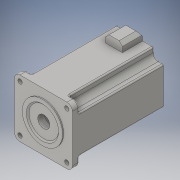
# Autodesk Inventor part: Body
Saved by Autodesk Inventor 2016 (Build 200138000, 138)
## iProperties
Created: 2017-05-16
Part Number: Body
Material: Generic
Document SubType Name: Modeling
Designer: M220404
Density: 1 g/cm^3
Appearance: Default
Author: M220404
Autodesk Inventor part; units mm, degrees
ref_plane "YZ Plane" through (0, 0, 0) normal (1, 0, 0) x (0, 1, 0)
ref_plane "XZ Plane" through (0, 0, 0) normal (0, 1, 0) x (-1, 0, 0)
ref_plane "XY Plane" through (0, 0, 0) normal (0, 0, 1) x (1, 0, 0)
sketch "Sketch1" plane through (0, 0, 0) normal (0, 0, 1) x (1, 0, 0)
  line L0 (0, 0) -> (86, 0)
  line L1 (86, 0) -> (86, 86)
  line L2 (86, 86) -> (0, 86)
  line L3 (0, 86) -> (0, 0)
  dimension "d0" = 86
  dimension "d1" = 86
  constraints: 8 end point, 2 parallel, 1 horizontal, 1 perpendicular
  measures "d0" distance of L2.end L1.end
  measures "d1" distance of L1.end L0.end
extrude "Extrusion1" add sketch "Sketch1" against normal blind 140
sketch "Sketch2" plane through (0, 0, 0) normal (0, 0, 1) x (1, 0, 0)
  line L0 (0, 86) -> (86, 86) construction
  line L1 (43, 86) -> (43, 0) construction
  line L2 (86, 0) -> (0, 0) construction
  line L3 (86, 86) -> (86, 0) construction
  line L4 (86, 43) -> (0, 43) construction
  line L5 (0, 0) -> (0, 86) construction
  circle A0 centre (43, 43) radius 30
  dimension "d5" = 60
  constraints: 5 midpoint, 4 end point, 1 centre point
  measures "d5" diameter of A0
extrude "Extrusion2" add sketch "Sketch2" along normal blind 1.5
sketch "Sketch3" plane through (43, 43, 1.5) normal (0, 0, 1) x (1, 0, 0)
  line L0 (43, 43) -> (-43, 43) construction
  line L1 (0, 43) -> (0, -43) construction
  line L2 (-43, -43) -> (43, -43) construction
  line L3 (43, -43) -> (43, 43) construction
  line L4 (43, 0) -> (-43, 0) construction
  line L5 (-43, 43) -> (-43, -43) construction
  circle A0 centre (0, 0) radius 30 projected
  circle A1 centre (0, 0) radius 7
  dimension "d8" = 14
  constraints: 4 end point, 4 midpoint, 1 centre point, 1 coincident
  measures "d8" diameter of A1
extrude "Extrusion3" add sketch "Sketch3" along normal blind 40 contours A1
hole "Hole1" at (43, 43, 41.5) direction (0, 0, -1) diameter 3 depth 13
ref_plane "Work Plane1" through (36, 43, 1.5) normal (1, 0, 0) x (0, 1, 0)
sketch "Sketch5" plane through (36, 43, 1.5) normal (1, 0, 0) x (0, 1, 0)
  line L0 (7, 40) -> (-7, 40) projected
  line L1 (-7, 0) -> (7, 0) projected
  line L2 (7, 0) -> (7, 40) projected
  line L3 (-7, 0) -> (-7, 40) projected
  line L4 (7, 40) -> (-7, 40) projected
  line L5 (-2.5, 17.5) -> (-2.5, 40)
  line L6 (-2.5, 40) -> (2.5, 40)
  line L7 (2.5, 40) -> (2.5, 17.5)
  line L8 (30, 0) -> (-30, 0) construction
  arc A0 (-2.5, 17.5) -> (2.5, 17.5) centre (0, 17.5) ccw
  point P0 (-43, -1.5)
  point P1 (0, 15)
  constraints: 6 end point, 3 point on circle, 1 centre point, 1 parallel, 1 point on line, 1 tangent
extrude "Extrusion4" cut sketch "Sketch5" along normal blind 2.438 contours L7 A0 L5 L0
sketch "Sketch6" plane through (0, 0, -140) normal (0, 0, -1) x (-1, 0, 0)
  circle A0 centre (-43, 43) radius 30 projected
  line L0 (-86, 86) -> (-71, 86)
  line L1 (-71, 86) -> (-71, 78.5)
  line L2 (-78.5, 71) -> (-86, 71)
  line L3 (-86, 71) -> (-86, 86)
  arc A1 (-78.5, 71) -> (-71, 78.5) centre (-78.5, 78.5) ccw
  line L4 (-86, 0) -> (-86, 15)
  line L5 (-86, 15) -> (-78.5, 15)
  line L6 (-71, 7.5) -> (-71, 0)
  line L7 (-71, 0) -> (-86, 0)
  arc A2 (-71, 7.5) -> (-78.5, 15) centre (-78.5, 7.5) ccw
  line L8 (0, 0) -> (-15, 0)
  line L9 (-15, 0) -> (-15, 7.5)
  line L10 (-7.5, 15) -> (0, 15)
  line L11 (0, 15) -> (0, 0)
  arc A3 (-7.5, 15) -> (-15, 7.5) centre (-7.5, 7.5) ccw
  line L12 (0, 86) -> (0, 71)
  line L13 (0, 71) -> (-7.5, 71)
  line L14 (-15, 78.5) -> (-15, 86)
  line L15 (-15, 86) -> (0, 86)
  arc A4 (-15, 78.5) -> (-7.5, 71) centre (-7.5, 78.5) ccw
  dimension "d71" = 15
  dimension "d72" = 15
  dimension "d75" = 360
  constraints: 32 end point, 8 point on circle, 4 centre point, 2 parallel, 1 horizontal, 1 perpendicular, 45 other
  measures "d71" distance of L2.end L0.start
  measures "d72" distance of L0.start L0.end
sketch "Sketch7" plane through (0, 0, 0) normal (0, 0, 1) x (1, 0, 0)
  circle A0 centre (8.2, 8.2) radius 3.25
  arc A1 (36.4617, 40.5) -> (36.4617, 45.5) centre (43, 43) ccw projected
  circle A2 centre (43, 43) radius 1.5 projected
  circle A3 centre (43, 43) radius 30 projected
  circle A4 centre (43, 43) radius 7 projected
  circle A5 centre (43, 43) radius 30 projected
  line L0 (86, 86) -> (0, 86) construction
  line L1 (43, 86) -> (43, 0) construction
  line L2 (0, 0) -> (86, 0) construction
  line L3 (0, 86) -> (0, 0) construction
  line L4 (0, 43) -> (86, 43) construction
  line L5 (86, 0) -> (86, 86) construction
  circle A6 centre (8.2, 77.8) radius 3.25
  circle A7 centre (77.8, 8.2) radius 3.25
  circle A8 centre (77.8, 77.8) radius 3.25
  dimension "d36" = 6.5
  dimension "d37" = 69.6
  dimension "d38" = 69.6
  constraints: 4 centre point, 4 end point, 4 midpoint, 3 symmetric about line, 3 other
  measures "d36" diameter of A0
  measures "d37" distance of A0.centre A6.centre
  measures "d38" distance of A8.centre A6.centre
extrude "Extrusion6" cut sketch "Sketch7" against normal through all contours A0 | A6 | A7 | A8
sketch "Sketch8" plane through (0, 86, 0) normal (0, 1, 0) x (1, 0, 0)
  line L0 (30.5, 135) -> (55.5, 135)
  line L1 (55.5, 135) -> (55.5, 105)
  line L2 (55.5, 105) -> (30.5, 105)
  line L3 (30.5, 105) -> (30.5, 135)
  line L4 (0, 140) -> (86, 140) projected
  line L5 (43, 135) -> (43, 105) construction
  point P0 (0, 0)
  point P1 (61, 140)
  dimension "d41" = 25
  dimension "d42" = 30
  dimension "d43" = 5
  constraints: 10 end point, 2 midpoint, 2 parallel, 1 horizontal, 1 perpendicular
  measures "d41" distance of L1.end L2.end
  measures "d42" distance of L0.end L1.end
  measures "d43" distance between parallel lines of L4 L0
extrude "Extrusion7" add sketch "Sketch8" along normal blind 13
chamfer "Chamfer1" distance 5 distance2 7 1 edges at (43, 99, -135) measured on face at (43, 99, -134.5)
fillet "Fillet1" radius 8 4 edges at (0, 86, -70) (86, 86, -70) (0, 0, -70) (86, 0, -70)
chamfer "Chamfer2" distance 5 angle 45 2 edges at (30.5, 99, -117.5) (55.5, 99, -117.5)
chamfer "Chamfer3" distance 1 angle 45 2 edges at (44.2711, 36.1164, 41.5) (44.2711, 49.8836, 41.5)
sketch "Sketch9" plane through (0, 0, -140) normal (0, 0, -1) x (-1, 0, 0)
  line L0 (0, 8) -> (0, 78) projected
  line L1 (-8, 86) -> (-78, 86) projected
  line L2 (-86, 78) -> (-86, 8) projected
  line L3 (-78, 0) -> (-8, 0) projected
  arc A0 (-86, 8) -> (-78, 0) centre (-78, 8) ccw projected
  arc A1 (-8, 0) -> (0, 8) centre (-8, 8) ccw projected
  arc A2 (0, 78) -> (-8, 86) centre (-8, 78) ccw projected
  arc A3 (-78, 86) -> (-86, 78) centre (-78, 78) ccw projected
  point P0 (0, 0)
extrude "Extrusion8" cut sketch "Sketch9" against normal blind 3
sketch "Sketch10" plane through (0, 0, -137) normal (0, 0, -1) x (-1, 0, 0)
  circle A0 centre (-43, 43) radius 1.5 projected
  circle A1 centre (-43, 43) radius 28
  point P0 (0, 0)
  dimension "d61" = 56
  constraints: 1 centre point, 1 coincident
  measures "d61" diameter of A1
extrude "Extrusion9" add sketch "Sketch10" along normal blind 3
chamfer "Chamfer4" distance 3 angle 45 1 edges at (71, 43, -140)
fillet "Fillet3" radius 2 4 edges at (86, 43, -137) (43, 86, -137) (0, 43, -137) (43, 0, -137)
extrude "Extrusion10" cut sketch "Sketch6" against normal blind 130 contours L0 L1 A1 L2 L3 | L4 L5 A2 L6 L7 | L8 L9 A3 L10 L11 | L12 L13 A4 L14 L15
fillet "Fillet4" radius 2 52 edges at (15, 85.4142, -136.4142) (15, 81.2501, -137) (12.8033, 73.1967, -137) (4.75, 71, -137) (0.5858, 71, -136.4142) (0, 71, -72.5001) (15, 86, -72.5001) (0, 74.5, -10) (11.5, 86, -10) (2.3431, 83.6569, -10) (0.5858, 15, -136.4142) (4.7499, 15, -137) (12.8033, 12.8033, -137) (15, 4.75, -137) (15, 0.5858, -136.4142) (15, 0, -72.5001) (0, 15, -72.5001) (11.5, 0, -10) (0, 11.5, -10) (2.3431, 2.3431, -10) (3.75, 15, -10) (15, 3.75, -10) (12.8033, 12.8033, -10) (15, 82.25, -10) (3.75, 71, -10) (12.8033, 73.1967, -10) (82.25, 71, -10) (71, 82.25, -10) (73.1967, 73.1967, -10) (74.5, 86, -10) (86, 74.5, -10) (83.6569, 83.6569, -10) (71, 85.4142, -136.4142) (71, 81.2501, -137) (73.1967, 73.1967, -137) (81.2501, 71, -137) (85.4142, 71, -136.4142) (86, 71, -72.5001) (71, 86, -72.5001) (86, 11.5, -10) (74.5, 0, -10) (83.6569, 2.3431, -10) (71, 3.75, -10) (82.25, 15, -10) (73.1967, 12.8033, -10) (85.4142, 15, -136.4142) (81.2501, 15, -137) (73.1967, 12.8033, -137) (71, 4.7499, -137) (71, 0.5858, -136.4142) (71, 0, -72.5001) (86, 15, -72.5001)
sketch "Sketch11" plane through (43, 43, 1.5) normal (0, 0, 1) x (1, 0, 0)
  circle A0 centre (0, 0) radius 30 projected
  circle A1 centre (0, 0) radius 22
  point P0 (-43, -43)
  dimension "d81" = 8
  constraints: 1 centre point
  measures "d81" radial gap between concentric circles of A0 A1
extrude "Extrusion11" cut sketch "Sketch11" against normal blind 2 contours A1
chamfer "Chamfer5" distance 2 angle 45 1 edges at (21, 43, 1.5) measured on face at (20.5, 43, 1.5)
sketch "Sketch13" plane through (43, 43, -0.5) normal (0, 0, 1) x (1, 0, 0)
  circle A0 centre (0, 0) radius 22 projected
  circle A1 centre (0, 0) radius 9
  circle A2 centre (0, 0) radius 1.5 projected
  circle A3 centre (0, 0) radius 7 projected
  circle A4 centre (0, 0) radius 1.5 projected
  circle A5 centre (0, 0) radius 7
  point P0 (-43, -43)
  dimension "d90" = 13
  constraints: 2 centre point, 1 coincident
  measures "d90" radial gap between concentric circles of A0 A1
extrude "Extrusion13" cut sketch "Sketch13" against normal blind 10 contours A1 | A2 | A3
sketch "Sketch14" plane through (43, 43, 41.5) normal (0, 0, 1) x (1, 0, 0)
  circle A0 centre (0, 0) radius 1.5 projected
  circle A1 centre (0, 0) radius 7
  point P0 (-43, -43)
  constraints: 1 centre point, 1 coincident
extrude "Extrusion14" cut sketch "Sketch14" against normal up to surface (52 mm away)
sketch "Sketch15" plane through (43, 43, 28.5) normal (0, 0, 1) x (1, 0, 0)
  circle A0 centre (0, 0) radius 1.5 projected
  circle A1 centre (0, 0) radius 1.5
  point P0 (-43, -43)
  constraints: 1 centre point, 1 coincident
extrude "Extrusion15" cut sketch "Sketch15" against normal up to surface (39 mm away)
body "Solid1"
